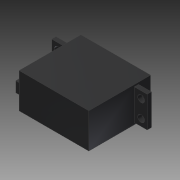
# Autodesk Inventor part: servo HK15138
Saved by Autodesk Inventor 2013 (Build 170138000, 138)
## iProperties
Created: 2014-04-23
Part Number: servo HK15138
Material: Generic
Document SubType Name: Modeling
Designer: Masta
Density: 1 g/cm^3
Author: Masta
Autodesk Inventor part; units mm, degrees
ref_plane "YZ Plane" through (0, 0, 0) normal (1, 0, 0) x (0, 1, 0)
ref_plane "XZ Plane" through (0, 0, 0) normal (0, 1, 0) x (-1, 0, 0)
ref_plane "XY Plane" through (0, 0, 0) normal (0, 0, 1) x (1, 0, 0)
sketch "Sketch1" plane through (0, 0, 0) normal (0, 0, 1) x (1, 0, 0)
  line L0 (0, 0) -> (40.6, 0)
  line L1 (40.6, 0) -> (40.6, 36)
  line L2 (40.6, 36) -> (0, 36)
  line L3 (0, 36) -> (0, 0)
  line L4 (0, 29) -> (-7.5, 29)
  line L5 (-7.5, 29) -> (-7.5, 26.5)
  line L6 (-7.5, 26.5) -> (0, 26.5)
  line L7 (0, 26.5) -> (0, 29)
  line L8 (40.6, 29) -> (48.1, 29)
  line L9 (48.1, 29) -> (48.1, 26.5)
  line L10 (48.1, 26.5) -> (40.6, 26.5)
  line L11 (40.6, 26.5) -> (40.6, 29)
  line L12 (0, 5) -> (-3, 5)
  line L13 (-3, 5) -> (-3, 1)
  line L14 (-3, 1) -> (0, 1)
  line L15 (0, 1) -> (0, 5)
  dimension "d0" = 40.6
  dimension "d1" = 36
  dimension "d2" = 7.5
  dimension "d3" = 2.5
  dimension "d4" = 7
  dimension "d5" = 3
  dimension "d6" = 4
  dimension "d7" = 1
  constraints: 32 end point, 8 parallel, 4 horizontal, 4 perpendicular, 3 collinear, 3 point on line
  measures "d0" distance of L2.end L1.end
  measures "d1" distance of L1.end L0.end
  measures "d2" distance of L6.end L5.end
  measures "d3" distance of L5.end L4.end
  measures "d4" distance between parallel lines of L2 L4
  measures "d5" distance of L14.end L13.end
  measures "d6" distance of L13.end L12.end
  measures "d7" distance between parallel lines of L0 L14
extrude "Extrusion1" add sketch "Sketch1" along normal mid plane 20.3 contours L3 L2 L1 L0
extrude "Extrusion2" add sketch "Sketch1" along normal mid plane 18 contours L1 L8 L9 L10 | L6 L5 L4 L3
extrude "Extrusion3" add sketch "Sketch1" along normal mid plane 6 contours L14 L13 L12 L3
sketch "Sketch2" plane through (-7.5, 29, 9) normal (0, 1, 0) x (1, 0, 0)
  line L0 (0, 18) -> (0, 0) projected
  line L1 (7.5, 18) -> (7.5, 0) projected
  line L2 (48.1, 0) -> (48.1, 18) projected
  line L3 (55.6, 0) -> (48.1, 0) projected
  line L4 (55.6, 18) -> (55.6, 0) projected
  line L5 (48.1, 18) -> (55.6, 18) projected
  line L6 (3.5, 14) -> (3.5, 4) construction
  line L7 (0, 9) -> (55.6, 9) construction
  line L8 (52.1, 14) -> (52.1, 4) construction
  line L9 (3.5, 4) -> (52.1, 4) construction
  line L10 (52.1, 14) -> (3.5, 14) construction
  point P0 (7.5, 9)
  dimension "d14" = 3.5
  dimension "d15" = 3.5
  dimension "d16" = 10
  constraints: 10 end point, 4 coincident, 3 perpendicular, 2 midpoint, 1 parallel, 1 symmetric about line
  measures "d14" distance between parallel lines of L0 L6
  measures "d15" distance between parallel lines of L4 L8
  measures "d16" distance of L8.start L8.end
hole "Hole1" at (-4, 29, -5) at (-4, 29, 5) at (44.6, 29, 5) at (44.6, 29, -5) direction (0, -1, 0) diameter 4 end through all
sketch "Sketch3" plane through (0, 36, 10.15) normal (0, 1, 0) x (1, 0, 0)
  line L0 (40.6, 20.3) -> (40.6, 0) projected
  line L1 (0, 20.3) -> (40.6, 20.3) projected
  circle A0 centre (30.6, 10.15) radius 7
  line L2 (0, 10.15) -> (30.6, 10.15) construction
  circle A1 centre (30.6, 10.15) radius 3
  dimension "d24" = 10
  dimension "d25" = 14
  dimension "d26" = 6
  constraints: 2 centre point, 2 end point, 1 coincident, 1 parallel
  measures "d24" distance from line of L0 L2.end
  measures "d25" diameter of A0
  measures "d26" diameter of A1
extrude "Extrusion4" add sketch "Sketch3" along normal blind 2
extrude "Extrusion5" add sketch "Sketch3" along normal blind 6 contours A1
chamfer "Chamfer1" distance 2 angle 45 1 edges at (23.6, 38, 0)
body "Solid1"
